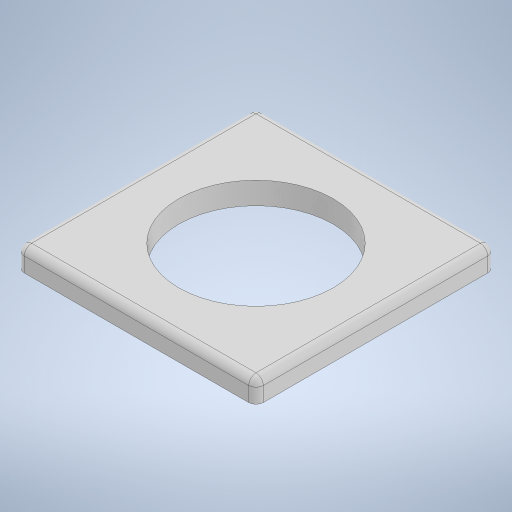
# Autodesk Inventor part: joystickBOXtop
Saved by Autodesk Inventor 2023 (Build 270158000, 158)
## iProperties
Created: 2023-09-26
Part Number: joystickBOXtop
Material: Generic
Document SubType Name: Modeling
Designer: Nikita
Density: 1 g/cm^3
Appearance: Default
Author: Nikita
Autodesk Inventor part; units mm, degrees
ref_plane "YZ Plane" through (0, 0, 0) normal (1, 0, 0) x (0, 1, 0)
ref_plane "XZ Plane" through (0, 0, 0) normal (0, 1, 0) x (-1, 0, 0)
ref_plane "XY Plane" through (0, 0, 0) normal (0, 0, 1) x (1, 0, 0)
sketch "Sketch1" plane through (0, 0, 0) normal (0, 1, 0) x (-1, 0, 0)
  line L0 (0, 0) -> (65, 0)
  line L1 (65, 0) -> (65, -65)
  line L2 (65, -65) -> (0, -65)
  line L3 (0, -65) -> (0, 0)
  dimension "d0" = 65
  dimension "d1" = 65
  constraints: 8 end point, 3 perpendicular, 1 horizontal
  measures "d0" distance of L0.start L0.end
  measures "d1" distance of L0.end L1.end
extrude "Extrusion1" add sketch "Sketch1" along normal blind 6
sketch "Sketch2" plane through (0, 6, 0) normal (0, 1, 0) x (1, 0, 0)
  line L0 (0, 0) -> (0, 65) construction
  line L1 (0, 65) -> (-65, 65) construction
  line L2 (0, 0) -> (-65, 65) construction
  line L3 (-65, 65) -> (-65, 0) construction
  line L4 (-65, 0) -> (0, 65) construction
  circle A0 centre (-32.5, 32.5) radius 21
  dimension "d4" = 42
  constraints: 6 end point, 2 perpendicular, 1 centre point, 1 midpoint
  measures "d4" diameter of A0
extrude "Extrusion2" cut sketch "Sketch2" against normal blind 6
fillet "Fillet1" radius 2 1 edges at (-32.5, 6, 0)
fillet "Fillet2" radius 2 3 edges at (0, 6, -33.5) (0, 5.4142, -0.5858) (0, 2, 0)
fillet "Fillet3" radius 2 3 edges at (-0.5858, 5.4142, -65) (0, 2, -65) (-33.5, 6, -65)
fillet "Fillet4" radius 2 5 edges at (-65, 5.4142, -0.5858) (-65, 2, 0) (-65, 5.4142, -64.4142) (-65, 2, -65) (-65, 6, -32.5)
body "Solid1"
